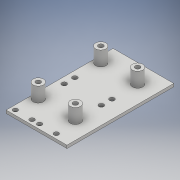
# Autodesk Inventor part: mountMount
Saved by Autodesk Inventor 2018 (Build 220112000, 112)
## iProperties
Created: 2018-05-09
Part Number: mountMount
Material: Generic
Document SubType Name: Modeling
Designer: s4321966
Density: 1 g/cm^3
Appearance: Default
Mass: 7.05449 g
Surface Area: 78.5664 cm^2
Volume: 7.05449 cm^3
Author: s4321966
Autodesk Inventor part; units mm, degrees
ref_plane "YZ Plane" through (0, 0, 0) normal (1, 0, 0) x (0, 1, 0)
ref_plane "XZ Plane" through (0, 0, 0) normal (0, 1, 0) x (-1, 0, 0)
ref_plane "XY Plane" through (0, 0, 0) normal (0, 0, 1) x (1, 0, 0)
sketch "Sketch1" plane through (0, 0, 0) normal (0, 0, 1) x (1, 0, 0)
  line L0 (0, 0) -> (41.5, 0)
  line L1 (41.5, 0) -> (41.5, -73)
  line L2 (41.5, -73) -> (0, -73)
  line L3 (0, -73) -> (0, 0)
  line L4 (0, -73) -> (3.11, -73)
  line L5 (0, -73) -> (3.11, -73) construction
  line L6 (3.11, -73) -> (3.11, -69.85)
  line L7 (3.11, -73) -> (6.26, -73) construction
  line L8 (3.11, -69.85) -> (14.54, -69.85)
  line L9 (14.54, -69.85) -> (19.65, -69.85)
  line L10 (19.65, -69.85) -> (31.08, -69.85)
  circle A0 centre (3.11, -69.85) radius 1.6
  circle A1 centre (14.54, -69.85) radius 1.6
  circle A2 centre (19.65, -69.85) radius 1.6
  circle A3 centre (31.08, -69.85) radius 1.6
  line L11 (3.11, -69.85) -> (3.11, -55.42)
  line L12 (3.11, -69.85) -> (17.54, -69.85) construction
  line L13 (0, -73) -> (4.33, -73)
  line L14 (0, -73) -> (4.33, -73) construction
  line L15 (4.33, -73) -> (4.33, -53.49)
  line L16 (3.11, -55.42) -> (6.6479, -55.42)
  circle A4 centre (4.33, -55.42) radius 1.651
  line L17 (4.33, -55.42) -> (4.33, -37.69)
  line L18 (4.33, -55.42) -> (22.06, -55.42) construction
  line L19 (4.33, -55.42) -> (29.68, -55.42)
  line L20 (4.33, -55.42) -> (29.68, -55.42) construction
  circle A5 centre (4.33, -37.69) radius 1.651
  circle A6 centre (29.68, -55.42) radius 1.651
  line L21 (4.33, -37.69) -> (39.0376, -37.69)
  line L22 (29.68, -55.42) -> (29.68, -25.3245)
  circle A7 centre (29.68, -37.69) radius 1.651
  line L23 (4.33, -37.69) -> (4.33, -30.44)
  line L24 (4.33, -37.69) -> (11.58, -37.69) construction
  line L25 (4.33, -30.44) -> (4.33, -12.71)
  line L26 (4.33, -30.44) -> (29.68, -30.44)
  line L27 (4.33, -30.44) -> (29.68, -30.44) construction
  line L28 (4.33, -12.71) -> (29.68, -12.71)
  circle A8 centre (29.48, -12.71) radius 1.651
  circle A9 centre (4.33, -12.71) radius 1.651
  circle A10 centre (4.33, -30.44) radius 1.651
  circle A11 centre (29.68, -30.44) radius 1.651
  dimension "d0" = 41.5
  dimension "d1" = 73
  dimension "d2" = 3.11
  dimension "d3" = 0
  dimension "d4" = 3.15
  dimension "d5" = 90
  dimension "d6" = 11.43
  dimension "d7" = 90
  dimension "d9" = 5.11
  dimension "d10" = 11.43
  dimension "d11" = 180
  dimension "d12" = 3.2
  dimension "d13" = 3.2
  dimension "d14" = 3.2
  dimension "d15" = 3.2
  dimension "d18" = 14.43
  dimension "d19" = 90
  dimension "d20" = 4.33
  dimension "d21" = 0
  dimension "d22" = 3.302
  dimension "d23" = 17.73
  dimension "d24" = 90
  dimension "d25" = 25.35
  dimension "d26" = 0
  dimension "d27" = 3.302
  dimension "d28" = 3.302
  dimension "d29" = 3.302
  dimension "d30" = 7.25
  dimension "d31" = 90
  dimension "d32" = 17.73
  dimension "d33" = 180
  dimension "d34" = 25.35
  dimension "d35" = 0
  dimension "d36" = 25.35
  dimension "d37" = 3.302
  dimension "d38" = 3.302
  dimension "d39" = 3.302
  dimension "d40" = 3.302
  constraints: 58 end point, 15 horizontal, 12 centre point, 9 coincident, 8 equal length, 5 perpendicular, 5 point on line, 4 vertical, 3 collinear, 2 parallel
  measures "d0" distance of L1.end L2.end
  measures "d1" distance of L0.end L1.end
  measures "d2" distance of L2.end L4.end
  measures "d3" distance between parallel lines of L4 L5
  measures "d4" distance of L4.end L6.end
  measures "d5" angle of L7 L6
  measures "d6" distance of L6.end L8.end
  measures "d7" angle of L6 L8
  measures "d9" distance of L8.end L9.end
  measures "d10" distance of L9.end L10.end
  measures "d11" angle of L10 L9
  measures "d12" diameter of A0
  measures "d13" diameter of A1
  measures "d14" diameter of A2
  measures "d15" diameter of A3
  measures "d18" distance of L11.start L11.end
  measures "d19" angle of L12 L11
  measures "d20" distance of L2.end L13.end
  measures "d21" distance between parallel lines of L13 L14
  measures "d22" diameter of A4
  measures "d23" distance of L17.start L17.end
  measures "d24" angle of L18 L17
  measures "d25" distance of L17.start L19.end
  measures "d26" distance between parallel lines of L19 L20
  measures "d27" diameter of A5
  measures "d28" diameter of A6
  measures "d29" diameter of A7
  measures "d30" distance of L21.start L23.end
  measures "d31" angle of L24 L23
  measures "d32" distance of L23.end L25.end
  measures "d33" angle of L25 L23
  measures "d34" distance of L23.end L26.end
  measures "d35" distance between parallel lines of L26 L27
  measures "d36" distance of L25.end L28.end
  measures "d37" diameter of A8
  measures "d38" diameter of A9
  measures "d39" diameter of A10
  measures "d40" diameter of A11
extrude "Extrusion2" add sketch "Sketch1" along normal blind 2 contours L0 L1 L2 L15 A0 A4 L16 L19 A6 L22 A7 A11 L26 A10 L23 A5 L17 L11 L6 L3 | L6 A0 L15 L2 | L11 A4 L15 A0 | L15 L17 A5 L21 A7 L22 A6 L19 L16 A4 | L23 A10 L26 A11 L22 A7 L21 A5
sketch "Sketch3" plane through (0, 0, 2) normal (0, 0, 1) x (1, 0, 0)
  circle A0 centre (4.33, -55.42) radius 1.651 projected
  circle A1 centre (4.33, -55.42) radius 3.5
  circle A2 centre (29.68, -55.42) radius 1.651 projected
  circle A3 centre (29.68, -55.42) radius 3.5
  circle A4 centre (4.33, -12.71) radius 1.651 projected
  circle A5 centre (4.33, -12.71) radius 3.5
  circle A6 centre (29.48, -12.71) radius 1.651 projected
  circle A7 centre (29.48, -12.71) radius 3.5
  point P0 (0, 0)
  dimension "d46" = 7
  dimension "d47" = 7
  dimension "d48" = 7
  dimension "d49" = 7
  constraints: 4 centre point, 4 coincident
  measures "d46" diameter of A1
  measures "d47" diameter of A3
  measures "d48" diameter of A5
  measures "d49" diameter of A7
extrude "Extrusion4" add sketch "Sketch3" along normal blind 10
body "Solid2"
